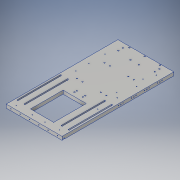
# Autodesk Inventor part: mplate
Saved by Autodesk Inventor 2019 (Build 230136000, 136)
## iProperties
Created: 2020-12-15
Part Number: mplate
Material: Aluminum 6061
Document SubType Name: Modeling
Designer: kananovicha
Density: 2.7 g/cm^3
Appearance: Aluminum - Flat
mp_hole_wid: 5.000 in
mp_hole_len: 7.000 in
mp_hole_l_offset: 18.800 in
mp_hole_w_offset: 6.000 in
mp_ts_v_margin: 1.800 in
mp_ts_h_margin: 0.856 in
ts_hole_h_spacing: 4.200 in
mp_len_loc: 24.000 in
mp_wid_loc: 12.000 in
mp_thick_loc: 0.750 in
mp_brahole_h_margin_loc: 0.500 in
mp_brahole_h_spacing_loc: 1.500 in
Author: kananovicha
Autodesk Inventor part; units mm, degrees
ref_plane "YZ Plane" through (0, 0, 0) normal (1, 0, 0) x (0, 1, 0)
ref_plane "XZ Plane" through (0, 0, 0) normal (0, 1, 0) x (-1, 0, 0)
ref_plane "XY Plane" through (0, 0, 0) normal (0, 0, 1) x (1, 0, 0)
sketch "Sketch1" plane through (0, 0, 0) normal (0, 0, 1) x (1, 0, 0)
  line L0 (-152.4, 9.525) -> (152.4, 9.525)
  line L1 (152.4, 9.525) -> (152.4, -9.525)
  line L2 (152.4, -9.525) -> (-152.4, -9.525)
  line L3 (-152.4, -9.525) -> (-152.4, 9.525)
  line L4 (-152.4, 9.525) -> (152.4, -9.525) construction
  line L5 (152.4, 9.525) -> (-152.4, -9.525) construction
  point P0 (0, 0)
  dimension "d0" = 304.8
  dimension "d1" = 19.05
  constraints: 12 end point, 2 midpoint, 2 parallel, 1 horizontal, 1 perpendicular
  measures "d0" distance of L1.end L2.end
  measures "d1" distance of L0.end L1.end
extrude "Extrusion1" add sketch "Sketch1" along normal blind 609.6
sketch "Sketch4" plane through (-152.4, 9.525, 0) normal (0, 1, 0) x (1, 0, 0)
  line L0 (215.9, -388.62) -> (88.9, -388.62)
  line L1 (88.9, -388.62) -> (88.9, -566.42)
  line L2 (88.9, -566.42) -> (215.9, -566.42)
  line L3 (215.9, -566.42) -> (215.9, -388.62)
  line L4 (215.9, -388.62) -> (88.9, -566.42) construction
  line L5 (88.9, -388.62) -> (215.9, -566.42) construction
  line L6 (0, 0) -> (0, -609.6) projected
  line L7 (0, 0) -> (304.8, 0) projected
  point P0 (152.4, 0)
  point P1 (152.4, -477.52)
  dimension "d18" = 127
  dimension "d19" = 177.8
  dimension "d20" = 152.4
  dimension "d24" = 477.52
  constraints: 12 end point, 2 midpoint, 2 parallel, 1 horizontal, 1 perpendicular
  measures "d18" distance of L2.end L1.end
  measures "d19" distance of L1.end L0.end
  measures "d20" distance from line of point (152.4, -477.52) L6
  measures "d24" distance from line of point (152.4, -477.52) L7
extrude "Extrusion2" cut sketch "Sketch4" against normal blind 304.8
sketch "Sketch7" plane through (152.4, -9.525, 0) normal (1, 0, 0) x (0, 0, -1)
  line L0 (0, 19.05) -> (-609.6, 19.05) projected
  point P0 (0, 9.525)
  point P1 (-76.2, 9.525)
  dimension "d39" = 76.2
  dimension "d40" = 9.525
  measures "d39" distance of point (-76.2, 9.525) point (0, 9.525)
  measures "d40" distance from line of L0 point (-76.2, 9.525)
hole "Hole5" at (152.4, 0, 76.2) direction (-1, 0, 0) diameter 4.9784 depth 33.02 tip angle 118 thread size "1/4-20 UNC" class "2B" standard "ANSI Unified Screw Threads"
sketch "Sketch8" plane through (152.4, -9.525, 0) normal (1, 0, 0) x (0, 0, -1)
  line L0 (0, 19.05) -> (0, 0) projected
  line L1 (0, 0) -> (-609.6, 0) projected
  circle A0 centre (-76.2, 9.525) radius 2.4892 projected
  line L2 (0, 19.05) -> (-609.6, 19.05) projected
  point P0 (0, 9.525)
  point P1 (-88.392, 10.541)
  dimension "d68" = 12.192
  dimension "d69" = 8.509
  measures "d68" horizontal distance of point (-88.392, 10.541) A0.centre
  measures "d69" distance from line of L2 point (-88.392, 10.541)
hole "Hole6" at (152.4, 1.016, 88.392) direction (-1, 0, 0) diameter 3.683 depth 14.9352 tip angle 118 thread size "10-24 UNC" class "2B" standard "ANSI Unified Screw Threads"
sketch "Sketch9" plane through (152.4, -9.525, 0) normal (1, 0, 0) x (0, 0, -1)
  line L0 (0, 19.05) -> (0, 0) projected
  line L1 (0, 19.05) -> (-609.6, 19.05) projected
  circle A0 centre (-76.2, 9.525) radius 2.4892 projected
  point P0 (0, 9.525)
  point P1 (-63.5, 10.795)
  dimension "d58" = 8.255
  dimension "d67" = 12.7
  measures "d58" distance from line of L1 point (-63.5, 10.795)
  measures "d67" horizontal distance of point (-63.5, 10.795) A0.centre
hole "Hole7" at (152.4, 1.27, 63.5) direction (-1, 0, 0) diameter 3.683 depth 14.9352 tip angle 118 thread size "10-24 UNC" class "2B" standard "ANSI Unified Screw Threads"
sketch "Sketch10" plane through (-152.4, -9.525, 0) normal (-1, 0, 0) x (0, 0, 1)
  line L0 (0, 0) -> (0, 19.05) projected
  line L1 (0, 19.05) -> (609.6, 19.05) projected
  point P0 (0, 9.525)
  point P1 (76.2, 9.525)
  dimension "d70" = 76.2
  dimension "d71" = 9.525
  measures "d70" distance from line of L0 point (76.2, 9.525)
  measures "d71" distance from line of L1 point (76.2, 9.525)
hole "Hole8" at (-152.4, 0, 76.2) direction (1, 0, 0) diameter 4.9784 depth 33.02 tip angle 118 thread size "1/4-20 UNC" class "2B" standard "ANSI Unified Screw Threads"
sketch "Sketch11" plane through (-152.4, -9.525, 0) normal (-1, 0, 0) x (0, 0, 1)
  circle A0 centre (76.2, 9.525) radius 2.4892 projected
  line L0 (0, 19.05) -> (609.6, 19.05) projected
  point P0 (0, 9.525)
  point P1 (88.392, 10.541)
  point P2 (63.5, 10.795)
  dimension "d79" = 12.192
  dimension "d80" = 8.509
  dimension "d81" = 12.7
  dimension "d82" = 8.255
  measures "d79" horizontal distance of A0.centre point (88.392, 10.541)
  measures "d80" distance from line of L0 point (88.392, 10.541)
  measures "d81" horizontal distance of A0.centre point (63.5, 10.795)
  measures "d82" distance from line of L0 point (63.5, 10.795)
hole "Hole9" at (-152.4, 1.016, 88.392) at (-152.4, 1.27, 63.5) direction (1, 0, 0) diameter 3.683 depth 14.9352 tip angle 118 thread size "10-24 UNC" class "2B" standard "ANSI Unified Screw Threads"
sketch "Sketch12" plane through (-152.4, -9.525, 0) normal (0, -1, 0) x (1, 0, 0)
  line L0 (304.8, 603.9485) -> (0, 603.9485)
  line L1 (0, 603.9485) -> (0, 594.4235)
  line L2 (0, 594.4235) -> (304.8, 594.4235)
  line L3 (304.8, 594.4235) -> (304.8, 603.9485)
  line L4 (304.8, 603.9485) -> (0, 594.4235) construction
  line L5 (0, 603.9485) -> (304.8, 594.4235) construction
  line L6 (0, 609.6) -> (304.8, 609.6) projected
  line L7 (304.8, 0) -> (304.8, 609.6) projected
  line L8 (0, 0) -> (0, 609.6) projected
  point P0 (152.4, 0)
  point P1 (152.4, 599.186)
  dimension "d91" = 10.414
  dimension "d92" = 9.525
  dimension "d93" = 0
  dimension "d94" = 0
  constraints: 12 end point, 2 midpoint, 2 parallel, 1 horizontal, 1 perpendicular
  measures "d91" distance from line of L6 point (152.4, 599.186)
  measures "d92" distance between parallel lines of L2 L0
  measures "d93" distance between parallel lines of L7 L3
  measures "d94" distance between parallel lines of L8 L1
extrude "Extrusion3" cut sketch "Sketch12" against normal blind 5.08 contours L3 L2 L1 L0
sketch "Sketch14" plane through (0, 0, 609.6) normal (0, 0, 1) x (1, 0, 0)
  line L0 (152.4, -9.525) -> (152.4, 9.525) projected
  line L1 (-152.4, -9.525) -> (152.4, -9.525) projected
  point P0 (0, 0)
  point P1 (127, 0)
  dimension "d113" = 25.4
  dimension "d114" = 9.525
  measures "d113" distance from line of point (127, 0) L0
  measures "d114" distance from line of L1 point (127, 0)
hole "Hole11" at (127, 0, 609.6) direction (0, 0, -1) diameter 3.683 depth 41.275 tip angle 118 thread size "10-24 UNC" class "2B" standard "ANSI Unified Screw Threads"
pattern_linear "Rectangular Pattern1" count 6 spacing 50.8 along (-1, 0, 0) of "Hole11"
sketch "Sketch16" plane through (-152.4, 9.525, 0) normal (0, 1, 0) x (1, 0, 0)
  line L0 (304.8, 0) -> (304.8, -609.6) projected
  line L1 (304.8, -609.6) -> (0, -609.6) projected
  point P0 (152.4, 0)
  point P1 (254, -558.8)
  point P2 (292.1, -558.8)
  point P3 (254, -325.12)
  point P4 (292.1, -325.12)
  dimension "d140" = 12.7
  dimension "d141" = 12.7
  dimension "d142" = 38.1
  dimension "d143" = 233.68
  dimension "d144" = 50.8
  dimension "d145" = 50.8
  dimension "d146" = 38.1
  dimension "d147" = 233.68
  measures "d140" distance from line of point (292.1, -558.8) L0
  measures "d141" distance from line of point (292.1, -325.12) L0
  measures "d142" distance of point (254, -325.12) point (292.1, -325.12)
  measures "d143" distance of point (292.1, -325.12) point (292.1, -558.8)
  measures "d144" distance from line of point (292.1, -558.8) L1
  measures "d145" distance from line of L1 point (254, -558.8)
  measures "d146" distance of point (292.1, -558.8) point (254, -558.8)
  measures "d147" distance of point (254, -325.12) point (254, -558.8)
hole "Hole13" at (101.6, 9.525, 558.8) at (139.7, 9.525, 558.8) at (101.6, 9.525, 325.12) at (139.7, 9.525, 325.12) direction (0, -1, 0) diameter 6.7564 end through all clearance for "Flat Head Machine Screw (82)" size "1/4" standard "Ansi Unified Screw Threads"
sketch "Sketch18" plane through (-152.4, 9.525, 0) normal (0, 1, 0) x (1, 0, 0)
  line L0 (288.7218, -325.12) -> (295.4782, -325.12)
  line L1 (295.4782, -325.12) -> (295.4782, -558.8)
  line L2 (295.4782, -558.8) -> (288.7218, -558.8)
  line L3 (288.7218, -558.8) -> (288.7218, -325.12)
  line L4 (288.7218, -325.12) -> (295.4782, -558.8) construction
  line L5 (295.4782, -325.12) -> (288.7218, -558.8) construction
  line L6 (304.8, -609.6) -> (0, -609.6) projected
  line L7 (304.8, 0) -> (304.8, -609.6) projected
  point P0 (152.4, 0)
  point P1 (292.1, -441.96)
  dimension "d161" = 6.7564
  dimension "d162" = 233.68
  dimension "d163" = 50.8
  dimension "d164" = 12.7
  constraints: 12 end point, 2 midpoint, 2 parallel, 1 horizontal, 1 perpendicular
  measures "d161" distance of L1.end L2.end
  measures "d162" distance of L2.end L0.start
  measures "d163" distance between parallel lines of L6 L2
  measures "d164" distance from line of L7 point (292.1, -441.96)
extrude "Extrusion5" cut sketch "Sketch18" against normal blind 19.05
pattern_linear "Rectangular Pattern3" count 2 spacing 38.1 along (-1, 0, 0) of "Extrusion5"
sketch "Sketch19" plane through (-152.4, 9.525, 0) normal (0, 1, 0) x (1, 0, 0)
  line L0 (304.8, -609.6) -> (0, -609.6) projected
  line L1 (0, 0) -> (0, -609.6) projected
  point P0 (152.4, 0)
  point P1 (12.7, -325.12)
  point P2 (12.7, -558.8)
  dimension "d173" = 50.8
  dimension "d175" = 12.7
  dimension "d177" = 12.7
  dimension "d179" = 233.68
  measures "d173" distance from line of L0 point (12.7, -558.8)
  measures "d175" distance from line of L1 point (12.7, -558.8)
  measures "d177" distance from line of L1 point (12.7, -325.12)
  measures "d179" distance of point (12.7, -325.12) point (12.7, -558.8)
hole "Hole14" at (-139.7, 9.525, 325.12) at (-139.7, 9.525, 558.8) direction (0, -1, 0) diameter 6.7564 end through all clearance for "Socket Head Cap Screw" size "1/4" standard "Ansi Unified Screw Threads"
sketch "Sketch20" plane through (-152.4, 9.525, 0) normal (0, 1, 0) x (1, 0, 0)
  line L0 (9.3218, -325.12) -> (16.0782, -325.12)
  line L1 (16.0782, -325.12) -> (16.0782, -558.8)
  line L2 (16.0782, -558.8) -> (9.3218, -558.8)
  line L3 (9.3218, -558.8) -> (9.3218, -325.12)
  line L4 (9.3218, -325.12) -> (16.0782, -558.8) construction
  line L5 (16.0782, -325.12) -> (9.3218, -558.8) construction
  line L6 (0, 0) -> (0, -609.6) projected
  line L7 (304.8, -609.6) -> (0, -609.6) projected
  point P0 (152.4, 0)
  point P1 (12.7, -441.96)
  dimension "d188" = 12.7
  dimension "d190" = 6.7564
  dimension "d191" = 50.8
  dimension "d192" = 233.68
  constraints: 12 end point, 2 midpoint, 2 parallel, 1 horizontal, 1 perpendicular
  measures "d188" distance from line of L6 point (12.7, -441.96)
  measures "d190" distance between parallel lines of L1 L3
  measures "d191" distance between parallel lines of L7 L2
  measures "d192" distance between parallel lines of L0 L2
extrude "Extrusion6" cut sketch "Sketch20" against normal blind 19.05
pattern_linear "Rectangular Pattern4" count 2 spacing 38.1 along (1, 0, 0) of "Hole14", "Extrusion6"
sketch "Sketch21" plane through (-152.4, 9.525, 0) normal (0, 1, 0) x (1, 0, 0)
  line L0 (304.8, 0) -> (304.8, -609.6) projected
  line L1 (0, 0) -> (304.8, 0) projected
  point P0 (152.4, 0)
  point P1 (273.05, -63.5)
  dimension "d198" = 31.75
  dimension "d200" = 63.5
  measures "d198" distance from line of L0 point (273.05, -63.5)
  measures "d200" distance from line of point (273.05, -63.5) L1
hole "Hole15" at (120.65, 9.525, 63.5) direction (0, -1, 0) diameter 3.683 end through all thread size "10-24 UNC" class "2B" standard "ANSI Unified Screw Threads"
pattern_linear "Rectangular Pattern5" count 4 spacing 106.68 along (0, 0, 1) of "Hole15"
pattern_linear "Rectangular Pattern6" count 4 spacing 71.12 along (0, 0, 1) of "Hole5", "Hole6", "Hole7"
pattern_linear "Rectangular Pattern7" count 4 spacing 71.12 along (0, 0, 1) of "Hole8", "Hole9"
sketch "Sketch22" plane through (-152.4, 9.525, 0) normal (0, 1, 0) x (1, 0, 0)
  line L0 (0, 0) -> (0, -609.6) projected
  line L1 (0, 0) -> (304.8, 0) projected
  point P0 (152.4, 0)
  point P1 (129.4, -60.8)
  dimension "d219" = 129.4
  dimension "d220" = 60.8
  measures "d219" distance from line of point (129.4, -60.8) L0
  measures "d220" distance from line of point (129.4, -60.8) L1
hole "Hole16" at (-23, 9.525, 60.8) direction (0, -1, 0) diameter 6.604 end through all clearance for "Socket Head Cap Screw" size "M6" standard "Ansi Metric M Profile"
pattern_linear "Rectangular Pattern8" count 2 spacing 46 along (1, 0, 0) of "Hole16"
sketch "Sketch23" plane through (-152.4, 9.525, 0) normal (0, 1, 0) x (1, 0, 0)
  line L0 (0, 0) -> (304.8, 0) projected
  line L1 (304.8, 0) -> (304.8, -609.6) projected
  point P0 (152.4, 0)
  point P1 (232.6, -145.8)
  dimension "d231" = 145.8
  dimension "d232" = 72.2
  measures "d231" distance from line of point (232.6, -145.8) L0
  measures "d232" distance from line of point (232.6, -145.8) L1
hole "Hole17" at (80.2, 9.525, 145.8) direction (0, -1, 0) diameter 5.5 end through all
pattern_linear "Rectangular Pattern9" count 2 spacing 30 along (-1, 0, 0) count 2 spacing 150 along (0, 0, 1) of "Hole17"
pattern_linear "Rectangular Pattern10" count 2 spacing 130.4 along (-1, 0, 0) of "Hole17", "Rectangular Pattern9"
sketch "Sketch24" plane through (-152.4, 9.525, 0) normal (0, 1, 0) x (1, 0, 0)
  line L0 (0, 0) -> (0, -609.6) projected
  circle A0 centre (129.4, -60.8) radius 3.302 projected
  point P0 (152.4, 0)
  point P1 (129.4, -353.5036)
  dimension "d249" = 129.4
  dimension "d250" = 292.7036
  measures "d249" distance from line of point (129.4, -353.504) L0
  measures "d250" distance of point (129.4, -353.504) A0.centre
hole "Hole18" at (-23, 9.525, 353.5036) direction (0, -1, 0) diameter 6.604 end through all clearance for "Socket Head Cap Screw" size "M6" standard "Ansi Metric M Profile"
pattern_linear "Rectangular Pattern11" count 2 spacing 46 along (1, 0, 0) count 2 spacing 13 along (0, 0, 1) of "Hole18"
sketch "Sketch25" plane through (-152.4, -9.525, 0) normal (0, -1, 0) x (1, 0, 0)
  line L0 (304.8, 0) -> (0, 0) projected
  line L1 (304.8, 0) -> (304.8, 594.4235) projected
  point P0 (152.4, 0)
  point P1 (152.4, 6.35)
  dimension "d264" = 6.35
  dimension "d265" = 152.4
  measures "d264" distance from line of point (152.4, 6.35) L0
  measures "d265" distance from line of point (152.4, 6.35) L1
hole "Hole19" at (0, -9.525, 6.35) direction (0, 1, 0) diameter 6.7564 end through all counterbore diameter 11.1252 counterbore depth 6.35 clearance for "Socket Head Cap Screw" size "1/4" standard "Ansi Unified Screw Threads"
sketch "Sketch26" plane through (-152.4, -9.525, 0) normal (0, -1, 0) x (1, 0, 0)
  line L0 (304.8, 0) -> (304.8, 594.4235) projected
  line L1 (304.8, 0) -> (0, 0) projected
  point P0 (152.4, 0)
  point P1 (236.22, 6.35)
  point P2 (68.58, 6.35)
  dimension "d273" = 68.58
  dimension "d274" = 167.64
  dimension "d275" = 6.35
  dimension "d276" = 6.35
  measures "d273" distance from line of point (236.22, 6.35) L0
  measures "d274" distance of point (68.58, 6.35) point (236.22, 6.35)
  measures "d275" distance from line of L1 point (68.58, 6.35)
  measures "d276" distance from line of L1 point (236.22, 6.35)
hole "Hole20" at (83.82, -9.525, 6.35) at (-83.82, -9.525, 6.35) direction (0, 1, 0) diameter 6.7564 end through all counterbore diameter 11.1252 counterbore depth 6.35 clearance for "Socket Head Cap Screw" size "1/4" standard "Ansi Unified Screw Threads"
sketch "Sketch27" plane through (-152.4, -9.525, 0) normal (0, -1, 0) x (1, 0, 0)
  line L0 (0, 0) -> (0, 594.4235) projected
  line L1 (304.8, 0) -> (304.8, 594.4235) projected
  line L2 (304.8, 0) -> (0, 0) projected
  point P0 (152.4, 0)
  point P1 (52.705, 25.4)
  point P2 (52.705, 50.8)
  point P3 (252.095, 50.8)
  point P4 (252.095, 25.4)
  dimension "mp_rb_offset_wid" = 52.705
  dimension "d285" = 52.705
  dimension "d286" = 52.705
  dimension "d287" = 52.705
  dimension "d288" = 25.4
  dimension "d289" = 25.4
  dimension "d290" = 25.4
  dimension "d291" = 25.4
  measures "mp_rb_offset_wid" distance from line of L0 point (52.705, 25.4)
  measures "d285" distance from line of L0 point (52.705, 50.8)
  measures "d286" distance from line of L1 point (252.095, 50.8)
  measures "d287" distance from line of L1 point (252.095, 25.4)
  measures "d288" distance from line of L2 point (52.705, 25.4)
  measures "d289" distance of point (52.705, 50.8) point (52.705, 25.4)
  measures "d290" distance of point (252.095, 50.8) point (252.095, 25.4)
  measures "d291" distance from line of L2 point (252.095, 25.4)
hole "Hole21" at (-99.695, -9.525, 25.4) at (-99.695, -9.525, 50.8) at (99.695, -9.525, 50.8) at (99.695, -9.525, 25.4) direction (0, 1, 0) diameter 6.7564 end through all counterbore diameter 11.1252 counterbore depth 6.35 clearance for "Socket Head Cap Screw" size "1/4" standard "Ansi Unified Screw Threads"
sketch "Sketch28" plane through (-152.4, 9.525, 0) normal (0, 1, 0) x (1, 0, 0)
  point P0 (152.4, 0)
  point P1 (267.1405, -586.4687)
  point P2 (190.7529, -588.9625)
  point P3 (122.0041, -588.9625)
  point P4 (33.6127, -588.9625)
  point P5 (33.02, -262.6378)
  point P6 (33.02, -191.1973)
  point P7 (33.02, -103.7768)
  point P8 (254.9556, -117.8769)
  point P9 (247.4356, -254.1777)
hole "Hole22" at (114.7405, 9.525, 586.4687) at (38.3529, 9.525, 588.9625) at (-30.3959, 9.525, 588.9625) at (-118.7873, 9.525, 588.9625) at (-119.38, 9.525, 262.6378) at (-119.38, 9.525, 191.1973) at (-119.38, 9.525, 103.7768) at (102.5556, 9.525, 117.8769) at (95.0356, 9.525, 254.1777) direction (0, -1, 0) diameter 3.302 depth 3.175 tip angle 118 thread size "8-32 UNC" class "2B" standard "ANSI Unified Screw Threads"
equation "\"d0\" = mp_wid_loc"
equation "\"d1\" = mp_thick_loc"
equation "\"d2\" = mp_len_loc"
equation "\"d18\" = mp_hole_wid"
equation "\"d19\" = mp_hole_len"
equation "\"d20\" = mp_hole_w_offset"
equation "\"d24\" = mp_hole_l_offset"
equation "\"d22\" = mp_wid_loc"
equation "\"d39\" = mp_mount_hole_l_offset"
equation "\"d40\" = mp_mount_hole_w_offset"
equation "\"d42\" = mp_camhole_depth_loc"
equation "\"d46\" = mp_camhole_depth_loc"
equation "\"d68\" = mp_secure_hole_l_offset"
equation "\"d69\" = mp_secure_hole_w_offset"
equation "\"d58\" = mp_secure_hole2_w_offset"
equation "\"d67\" = mp_secure_hole2_l_offset"
equation "\"d70\" = mp_mount_hole_l_offset"
equation "\"d71\" = mp_mount_hole_w_offset"
equation "\"d73\" = mp_camhole_depth_loc"
equation "\"d77\" = mp_camhole_depth_loc"
equation "\"d79\" = mp_secure_hole_l_offset"
equation "\"d80\" = mp_secure_hole_w_offset"
equation "\"d81\" = mp_secure_hole2_l_offset"
equation "\"d82\" = mp_secure_hole2_w_offset"
equation "\"d91\" = mp_grove_offset"
equation "\"d92\" = mp_grove_width"
equation "\"d95\" = mp_grove_depth"
equation "\"d113\" = mp_hingeHole_horMargin_loc"
equation "\"d114\" = mp_hingeHole_vertMargin_loc"
equation "\"d116\" = mp_hinge_hole_depth"
equation "\"d124\" = mp_hingeHole_spacing_loc"
equation "\"d140\" = mp_brahole_h_margin_loc"
equation "\"d141\" = mp_brahole_h_margin_loc"
equation "\"d142\" = mp_brahole_h_spacing_loc"
equation "\"d143\" = mp_brahole_v_spacing"
equation "\"d144\" = mp_brahole_v_margin"
equation "\"d145\" = mp_brahole_v_margin"
equation "\"d146\" = mp_brahole_h_spacing_loc"
equation "\"d147\" = mp_brahole_v_spacing"
equation "\"d153\" = mp_brahole_depth_nut"
equation "\"d161\" = mp_brahole_smallDiam"
equation "\"d162\" = mp_brahole_v_spacing"
equation "\"d163\" = mp_brahole_v_margin"
equation "\"d164\" = mp_brahole_h_margin_loc"
equation "\"d165\" = mp_thick_loc"
equation "\"d172\" = mp_brahole_h_spacing_loc"
equation "\"d173\" = mp_brahole_v_margin"
equation "\"d175\" = mp_brahole_h_margin_loc"
equation "\"d177\" = mp_brahole_h_margin_loc"
equation "\"d179\" = mp_brahole_v_spacing"
equation "\"d188\" = mp_brahole_h_margin_loc"
equation "\"d190\" = mp_brahole_smallDiam"
equation "\"d191\" = mp_brahole_v_margin"
equation "\"d192\" = mp_brahole_v_spacing"
equation "\"d193\" = mp_thick_loc"
equation "\"d197\" = mp_brahole_h_spacing_loc"
equation "\"d198\" = mp_ts_hole_h_margin"
equation "\"d200\" = mp_ts_hole_v_margin"
equation "\"d211\" = ts_hole_h_spacing"
equation "\"d214\" = mp_brahole_pattern_dispacement"
equation "\"d217\" = mp_brahole_pattern_dispacement"
equation "\"d219\" = mp_bf_mountHole_hor_offset"
equation "\"d220\" = mp_bf_mountHole_vert_offset"
equation "\"d230\" = bf12_dim_p"
equation "\"d231\" = mp_brm_hole_v_offset"
equation "\"d232\" = mp_brm_hole_h_offset"
equation "\"d233\" = brm_hole_diam"
equation "\"d242\" = brm_hole_h_spacing"
equation "\"d245\" = brm_hole_v_spacing"
equation "\"d248\" = brm_h_spacing"
equation "\"d249\" = mp_bf_mountHole_hor_offset"
equation "\"d250\" = mp_bk_mountHole_hor_spacing"
equation "\"d260\" = bf12_dim_p"
equation "\"d263\" = bk_hole_v_spacing"
equation "\"d264\" = 0.5 * smp_thi"
equation "\"d265\" = 0.5 * mp_wid"
equation "\"d273\" = 0.5 * mp_wid - 0.5 * smp_wid + smp_mhole_margin"
equation "\"d274\" = smp_wid - 2 * smp_mhole_margin"
equation "\"d275\" = 0.5 * smp_thi"
equation "\"d276\" = 0.5 * smp_thi"
equation "\"mp_rb_offset_wid\" = 0.5 * mp_wid - 0.5 * smp_wid + 0.5 * rb_thi"
equation "\"d285\" = mp_rb_offset_wid"
equation "\"d286\" = mp_rb_offset_wid"
equation "\"d287\" = mp_rb_offset_wid"
equation "\"d288\" = mp_rb_offset_len"
equation "\"d289\" = mp_rb_hole_spacing"
equation "\"d290\" = mp_rb_hole_spacing"
equation "\"d291\" = mp_rb_offset_len"
equation "\"mp_len_loc\" = mp_len"
equation "\"mp_wid_loc\" = mp_wid"
equation "\"mp_thick_loc\" = mp_thick"
equation "\"mp_hole_wid\" = 127"
equation "\"mp_hole_len\" = 177.8"
equation "\"mp_hole_w_offset\" = 0.5 * mp_wid_loc + 0 * mp_hole_wid"
equation "\"test\" = 25.4"
equation "\"mp_secure_hole_l_offset\" = 12.192"
equation "\"mp_secure_hole2_l_offset\" = 12.7"
equation "\"mp_mount_hole_l_offset\" = 76.2"
equation "\"mp_mount_hole_w_offset\" = 0.5 * mp_thick_loc"
equation "\"mp_grove_offset\" = 10.414"
equation "\"mp_grove_width\" = 9.525"
equation "\"mp_grove_depth\" = 5.08"
equation "\"mp_hingeHole_horMargin_loc\" = mp_hingeHole_horMargin"
equation "\"mp_hingeHole_vertMargin_loc\" = mp_hingeHole_vertMargin"
equation "\"mp_hingeHole_spacing_loc\" = mp_hingeHole_spacing"
equation "\"mp_brahole_h_margin_loc\" = mp_brahole_h_margin"
equation "\"mp_brahole_h_spacing_loc\" = mp_brahole_h_spacing"
equation "\"mp_brahole_v_margin\" = 50.8"
equation "\"mp_brahole_v_spacing\" = 233.68"
equation "\"mp_brahole_depth_nut\" = 5.5626"
equation "\"mp_brahole_diam\" = 11.50937"
equation "\"mp_brahole_smallDiam\" = 6.7564"
equation "\"mp_ts_hole_h_margin\" = 0.5 * mp_brahole_h_spacing_loc + mp_brahole_h_margin_loc"
equation "\"mp_ts_v_margin\" = 45.72"
equation "\"mp_ts_hole_v_margin\" = mp_ts_v_margin + ts_hole_h_margin"
equation "\"mp_brahole_pattern_dispacement\" = 71.12"
equation "\"mp_bf_mountHole_hor_offset\" = 0.5 * mp_wid_loc - 0.5 * bf12_dim_p"
equation "\"mp_brm_hole_v_offset\" = brm_hole_v_offset + brm_v_offset"
equation "\"mp_brm_hole_h_offset\" = brm_hole_h_offset + brm_h_offset"
equation "\"mp_rb_offset_len\" = rb_bhole_long_margin + smp_thi"
equation "\"mp_rb_hole_spacing\" = rb_len - 2 * rb_bhole_long_margin"
equation "\"mp_camhole_depth_loc\" = mp_camhole_depth"
equation "\"mp_hinge_hole_depth\" = 38.1"
equation "\"ts_hole_h_spacing\" = 106.68"
equation "\"bf12_dim_p\" = 46"
equation "\"brm_hole_diam\" = 5.5"
equation "\"brm_hole_h_spacing\" = 30"
equation "\"brm_hole_v_spacing\" = 150"
equation "\"brm_h_spacing\" = 130.4"
equation "\"bk_hole_v_spacing\" = 13"
equation "\"mp_len\" = 609.6"
equation "\"mp_wid\" = 304.8"
equation "\"mp_thick\" = 19.05"
equation "\"mp_hingeHole_horMargin\" = 25.4"
equation "\"mp_hingeHole_vertMargin\" = 9.525"
equation "\"mp_hingeHole_spacing\" = 50.8"
equation "\"mp_brahole_h_margin\" = 12.7"
equation "\"mp_brahole_h_spacing\" = 38.1"
equation "\"ts_hole_h_margin\" = 17.78"
equation "\"brm_hole_v_offset\" = 75"
equation "\"brm_v_offset\" = 70.8"
equation "\"brm_hole_h_offset\" = 7.5"
equation "\"brm_h_offset\" = 64.7"
equation "\"rb_bhole_long_margin\" = 12.7"
equation "\"smp_thi\" = 12.7"
equation "\"rb_len\" = 50.8"
equation "\"mp_camhole_depth\" = 33.02"
equation "\"mp_hole_l_offset\" = 477.52"
equation "\"mp_secure_hole_w_offset\" = 8.509"
equation "\"mp_secure_hole2_w_offset\" = 8.255"
equation "\"mp_bf_mountHole_vert_offset\" = 60.8"
equation "\"mp_bk_mountHole_hor_spacing\" = 292.7036"
equation "\"smp_wid\" = 218.44"
equation "\"smp_mhole_margin\" = 25.4"
equation "\"rb_thi\" = 19.05"
body "Solid1"
